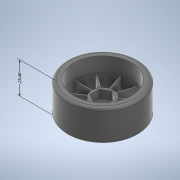
# Autodesk Inventor part: wheel
Saved by Autodesk Inventor 2022 (Build 260153000, 153)
## iProperties
Created: 2023-03-17
Part Number: wheel
Material: 一般
Document SubType Name: Modeling
Designer: JOU
Density: 1 g/cm^3
Appearance: 預設
Author: JOU
Autodesk Inventor part; units mm, degrees
ref_plane "YZ Plane" through (0, 0, 0) normal (1, 0, 0) x (0, 1, 0)
ref_plane "XZ Plane" through (0, 0, 0) normal (0, 1, 0) x (-1, 0, 0)
ref_plane "XY Plane" through (0, 0, 0) normal (0, 0, 1) x (1, 0, 0)
sketch "草圖1" plane through (0, 0, 0) normal (0, 1, 0) x (-1, 0, 0)
  circle A0 centre (0, 0) radius 26
  dimension "d0" = 52
  constraints: 1 centre point, 1 coincident
  measures "d0" diameter of A0
extrude "擠出1" add sketch "草圖1" along normal blind 23
fillet "圓角1" radius 2 2 edges at (26, 23, 0) (26, 0, 0)
sketch "草圖2" plane through (0, 23, 0) normal (0, 1, 0) x (1, 0, 0)
  circle A0 centre (0, 0) radius 21
  dimension "d4" = 42
  constraints: 1 centre point, 1 coincident
  measures "d4" diameter of A0
extrude "擠出2" cut sketch "草圖2" against normal blind 11
sketch "草圖3" plane through (0, 12, 0) normal (0, 1, 0) x (1, 0, 0)
  circle A0 centre (0, 0) radius 8
  line L0 (-6, 3.4641) -> (0, 6.9282)
  line L1 (0, 6.9282) -> (6, 3.4641)
  line L2 (6, 3.4641) -> (6, -3.4641)
  line L3 (6, -3.4641) -> (0, -6.9282)
  line L4 (0, -6.9282) -> (-6, -3.4641)
  line L5 (-6, -3.4641) -> (-6, 3.4641)
  dimension "d7" = 12
  dimension "d8" = 16
  constraints: 12 end point, 2 coincident, 1 centre point, 1 vertical, 13 other
  measures "d7" distance between parallel lines of L2 L5
  measures "d8" diameter of A0
extrude "擠出3" cut sketch "草圖3" against normal blind 6 contours L0 L1 L2 L3 L4 L5
sketch "草圖4" plane through (0, 12, 0) normal (0, 1, 0) x (1, 0, 0)
  circle A0 centre (0, 0) radius 21 projected
  circle A1 centre (0, 0) radius 8 projected
  line L0 (0, 0) -> (-21, 0)
  line L1 (0, 0) -> (-16.9894, 12.3435)
  circle A2 centre (0, 0) radius 21 projected
  line L2 (-21, 0.5) -> (-1.5388, 0.5)
  line L3 (-1.5388, 0.5) -> (-17.2832, 11.939)
  circle A3 centre (0, 0) radius 20.5
  point P0 (-16.8738, 11.6415)
  point P1 (-20.4939, 0.5)
  point P2 (-7.9844, 0.5)
  point P3 (-6.7534, 4.2886)
  dimension "d11" = 36
  dimension "d12" = 0.5
  dimension "d13" = 0.5
  constraints: 8 end point, 1 centre point, 1 horizontal, 1 horizontal alignment, 1 point on circle, 2 other
  measures "d11" angle of L1 L0
  measures "d12" distance between parallel lines of L0 L2
extrude "擠出4" cut sketch "草圖4" against normal through all contours L3 A1 L2 A3
pattern_circular "環形陣列1" count 10 over 360 about axis through (0, -10, 0) along (0, 1, 0) of "擠出4"
sketch "草圖5" plane through (0, 6, 0) normal (0, 1, 0) x (1, 0, 0)
  circle A0 centre (0, 0) radius 2
  dimension "d19" = 4
  constraints: 1 centre point, 1 coincident
  measures "d19" diameter of A0
extrude "擠出5" cut sketch "草圖5" against normal through all
sketch "草圖6" plane through (0, 23, 0) normal (0, 1, 0) x (1, 0, 0)
  circle A0 centre (0, 0) radius 26 projected
  line L0 (48.5339, -26) -> (-4.5845, -26)
  line L1 (-4.5845, -26) -> (-136.2974, 21.9396)
  line L2 (0, 0) -> (-8.8925, -24.432)
  line L3 (0, 36.4) -> (0, -36.4) projected
  line L4 (4.5845, -26) -> (40.2795, -13.0081)
  dimension "d22" = 20
  dimension "d23" = 20
  constraints: 8 end point, 2 horizontal, 2 point on line, 4 other
  measures "d22" angle of L0 L1
  measures "d23" angle of L0 L4
